Autodesk Fusion 360 part; units mm, degrees
(part 13 of 15)
  spline S115 degree 5 poles (45.7907, -108.2568) (45.7949, -108.2665) (45.806, -108.2927) (45.8241, -108.3354) (45.849, -108.3946) (45.8806, -108.4705) (45.9146, -108.5534) (45.9483, -108.6365) (45.9816, -108.7198) (46.0145, -108.8033) (46.0471, -108.8871) (46.0794, -108.971) (46.1114, -109.0551) (46.143, -109.1395) (46.1743, -109.224) (46.2052, -109.3087) (46.2359, -109.3936) (46.2662, -109.4787) (46.2962, -109.564) (46.3259, -109.6495) (46.3553, -109.7351) (46.3844, -109.8209) (46.4132, -109.9069) (46.4417, -109.9931) (46.4699, -110.0794) (46.4977, -110.1659) (46.5253, -110.2526) (46.5526, -110.3394) (46.5796, -110.4264) (46.6063, -110.5136) (46.6328, -110.6009) (46.6589, -110.6884) (46.6848, -110.776) (46.7103, -110.8637) (46.7356, -110.9517) (46.7606, -111.0397) (46.7854, -111.128) (46.8098, -111.2163) (46.834, -111.3048) (46.8579, -111.3935) (46.8816, -111.4823) (46.9049, -111.5712) (46.928, -111.6603) (46.9463, -111.7317) (46.9599, -111.7853) (46.9689, -111.821) (46.9733, -111.8389) knots 0.405839 0.405839 0.405839 0.405839 0.405839 0.405839 0.414286 0.428571 0.442857 0.457143 0.471429 0.485714 0.5 0.514286 0.528571 0.542857 0.557143 0.571429 0.585714 0.6 0.614286 0.628571 0.642857 0.657143 0.671429 0.685714 0.7 0.714286 0.728571 0.742857 0.757143 0.771429 0.785714 0.8 0.814286 0.828571 0.842857 0.857143 0.871429 0.885714 0.9 0.914286 0.928571 0.942857 0.957143 0.971429 0.985714 1 1 1 1 1 1
  arc A115 (45.9144, -112.6316) -> (46.9733, -111.8389) centre (2.0032, -52.8695) ccw
  spline S116 degree 5 poles (45.9144, -112.6316) (45.8985, -112.6223) (45.8667, -112.6036) (45.8191, -112.5754) (45.7558, -112.5378) (45.6769, -112.4906) (45.5981, -112.4431) (45.5196, -112.3954) (45.4412, -112.3475) (45.3631, -112.2993) (45.2852, -112.251) (45.2075, -112.2024) (45.1301, -112.1536) (45.0529, -112.1045) (44.9758, -112.0553) (44.8991, -112.0058) (44.8225, -111.956) (44.7462, -111.9061) (44.6701, -111.8559) (44.5942, -111.8055) (44.5186, -111.7548) (44.4432, -111.7039) (44.3681, -111.6528) (44.2932, -111.6015) (44.2185, -111.5499) (44.1441, -111.498) (44.07, -111.4459) (43.9961, -111.3936) (43.9224, -111.341) (43.8491, -111.2882) (43.776, -111.2351) (43.7031, -111.1818) (43.6306, -111.1282) (43.5583, -111.0744) (43.4863, -111.0203) (43.4145, -110.9659) (43.3431, -110.9113) (43.2719, -110.8564) (43.2011, -110.8012) (43.1305, -110.7458) (43.0603, -110.6901) (42.9903, -110.6341) (42.9264, -110.5825) (42.8766, -110.5419) (42.8407, -110.5125) (42.8188, -110.4944) (42.8106, -110.4877) knots -1 -1 -1 -1 -1 -1 -0.985714 -0.971429 -0.957143 -0.942857 -0.928571 -0.914286 -0.9 -0.885714 -0.871429 -0.857143 -0.842857 -0.828571 -0.814286 -0.8 -0.785714 -0.771429 -0.757143 -0.742857 -0.728571 -0.714286 -0.7 -0.685714 -0.671429 -0.657143 -0.642857 -0.628571 -0.614286 -0.6 -0.585714 -0.571429 -0.557143 -0.542857 -0.528571 -0.514286 -0.5 -0.485714 -0.471429 -0.457143 -0.442857 -0.428571 -0.414286 -0.405839 -0.405839 -0.405839 -0.405839 -0.405839 -0.405839
  arc A116 (41.7279, -111.2395) -> (42.8106, -110.4877) centre (2.0032, -52.8695) ccw
  spline S117 degree 5 poles (41.7279, -111.2395) (41.7313, -111.2494) (41.7406, -111.2763) (41.7556, -111.3202) (41.7762, -111.381) (41.8023, -111.459) (41.8303, -111.5441) (41.8579, -111.6294) (41.8852, -111.7149) (41.9121, -111.8005) (41.9387, -111.8864) (41.9649, -111.9724) (41.9907, -112.0586) (42.0163, -112.145) (42.0414, -112.2316) (42.0663, -112.3183) (42.0908, -112.4051) (42.115, -112.4922) (42.1388, -112.5794) (42.1624, -112.6668) (42.1856, -112.7543) (42.2085, -112.842) (42.231, -112.9298) (42.2533, -113.0178) (42.2753, -113.1059) (42.2969, -113.1942) (42.3182, -113.2826) (42.3393, -113.3711) (42.36, -113.4598) (42.3804, -113.5487) (42.4005, -113.6376) (42.4204, -113.7267) (42.4399, -113.816) (42.4592, -113.9054) (42.4781, -113.9949) (42.4968, -114.0845) (42.5152, -114.1742) (42.5332, -114.2641) (42.5511, -114.3541) (42.5686, -114.4443) (42.5858, -114.5345) (42.6028, -114.6249) (42.6195, -114.7154) (42.6326, -114.7879) (42.6423, -114.8423) (42.6487, -114.8786) (42.6519, -114.8968) knots 0.405839 0.405839 0.405839 0.405839 0.405839 0.405839 0.414286 0.428571 0.442857 0.457143 0.471429 0.485714 0.5 0.514286 0.528571 0.542857 0.557143 0.571429 0.585714 0.6 0.614286 0.628571 0.642857 0.657143 0.671429 0.685714 0.7 0.714286 0.728571 0.742857 0.757143 0.771429 0.785714 0.8 0.814286 0.828571 0.842857 0.857143 0.871429 0.885714 0.9 0.914286 0.928571 0.942857 0.957143 0.971429 0.985714 1 1 1 1 1 1
  arc A117 (41.5391, -115.6119) -> (42.6519, -114.8968) centre (2.0032, -52.8695) ccw
  spline S118 degree 5 poles (41.5391, -115.6119) (41.524, -115.6015) (41.4936, -115.5806) (41.4481, -115.5491) (41.3876, -115.5071) (41.3123, -115.4543) (41.2371, -115.4013) (41.1622, -115.3481) (41.0875, -115.2947) (41.013, -115.2412) (40.9387, -115.1874) (40.8647, -115.1334) (40.7909, -115.0791) (40.7174, -115.0247) (40.6441, -114.9701) (40.571, -114.9152) (40.4982, -114.8602) (40.4256, -114.8049) (40.3533, -114.7494) (40.2812, -114.6937) (40.2094, -114.6378) (40.1379, -114.5817) (40.0666, -114.5253) (39.9955, -114.4687) (39.9247, -114.412) (39.8542, -114.3549) (39.784, -114.2977) (39.714, -114.2402) (39.6443, -114.1825) (39.5749, -114.1246) (39.5058, -114.0664) (39.4369, -114.008) (39.3684, -113.9494) (39.3001, -113.8906) (39.2321, -113.8315) (39.1645, -113.7721) (39.0971, -113.7126) (39.03, -113.6527) (38.9633, -113.5927) (38.8969, -113.5323) (38.8308, -113.4718) (38.765, -113.4109) (38.7049, -113.3549) (38.6581, -113.3108) (38.6245, -113.279) (38.6038, -113.2594) (38.5962, -113.2521) knots -1 -1 -1 -1 -1 -1 -0.985714 -0.971429 -0.957143 -0.942857 -0.928571 -0.914286 -0.9 -0.885714 -0.871429 -0.857143 -0.842857 -0.828571 -0.814286 -0.8 -0.785714 -0.771429 -0.757143 -0.742857 -0.728571 -0.714286 -0.7 -0.685714 -0.671429 -0.657143 -0.642857 -0.628571 -0.614286 -0.6 -0.585714 -0.571429 -0.557143 -0.542857 -0.528571 -0.514286 -0.5 -0.485714 -0.471429 -0.457143 -0.442857 -0.428571 -0.414286 -0.405839 -0.405839 -0.405839 -0.405839 -0.405839 -0.405839
  arc A118 (37.4626, -113.9247) -> (38.5962, -113.2521) centre (2.0032, -52.8695) ccw
  spline S119 degree 5 poles (37.4626, -113.9247) (37.4653, -113.9349) (37.4726, -113.9624) (37.4845, -114.0072) (37.5007, -114.0693) (37.5211, -114.149) (37.543, -114.2358) (37.5645, -114.3229) (37.5856, -114.4101) (37.6063, -114.4975) (37.6267, -114.585) (37.6467, -114.6727) (37.6663, -114.7605) (37.6856, -114.8485) (37.7046, -114.9366) (37.7232, -115.0249) (37.7414, -115.1133) (37.7593, -115.2018) (37.7769, -115.2905) (37.7942, -115.3793) (37.8111, -115.4683) (37.8276, -115.5574) (37.8439, -115.6466) (37.8598, -115.7359) (37.8754, -115.8254) (37.8907, -115.915) (37.9057, -116.0047) (37.9204, -116.0945) (37.9347, -116.1845) (37.9487, -116.2745) (37.9625, -116.3647) (37.9759, -116.455) (37.989, -116.5454) (38.0018, -116.6359) (38.0144, -116.7266) (38.0266, -116.8173) (38.0385, -116.9081) (38.0501, -116.9991) (38.0615, -117.0901) (38.0725, -117.1813) (38.0833, -117.2726) (38.0938, -117.3639) (38.1039, -117.4554) (38.1119, -117.5286) (38.1177, -117.5836) (38.1215, -117.6203) (38.1234, -117.6386) knots 0.405839 0.405839 0.405839 0.405839 0.405839 0.405839 0.414286 0.428571 0.442857 0.457143 0.471429 0.485714 0.5 0.514286 0.528571 0.542857 0.557143 0.571429 0.585714 0.6 0.614286 0.628571 0.642857 0.657143 0.671429 0.685714 0.7 0.714286 0.728571 0.742857 0.757143 0.771429 0.785714 0.8 0.814286 0.828571 0.842857 0.857143 0.871429 0.885714 0.9 0.914286 0.928571 0.942857 0.957143 0.971429 0.985714 1 1 1 1 1 1
  arc A119 (36.9624, -118.2725) -> (38.1234, -117.6386) centre (2.0032, -52.8695) ccw
  spline S120 degree 5 poles (36.9624, -118.2725) (36.948, -118.261) (36.9192, -118.238) (36.8761, -118.2034) (36.8188, -118.1571) (36.7474, -118.0991) (36.6762, -118.0409) (36.6052, -117.9825) (36.5345, -117.9239) (36.464, -117.8652) (36.3938, -117.8062) (36.3238, -117.7471) (36.2541, -117.6877) (36.1846, -117.6282) (36.1154, -117.5685) (36.0465, -117.5086) (35.9778, -117.4484) (35.9093, -117.3881) (35.8411, -117.3276) (35.7732, -117.2669) (35.7056, -117.206) (35.6382, -117.1449) (35.5711, -117.0836) (35.5043, -117.0221) (35.4377, -116.9604) (35.3715, -116.8985) (35.3055, -116.8364) (35.2398, -116.7741) (35.1744, -116.7116) (35.1093, -116.6489) (35.0445, -116.5859) (34.98, -116.5228) (34.9158, -116.4594) (34.8519, -116.3958) (34.7883, -116.332) (34.725, -116.268) (34.6621, -116.2038) (34.5995, -116.1393) (34.5372, -116.0746) (34.4752, -116.0097) (34.4136, -115.9446) (34.3524, -115.8792) (34.2964, -115.819) (34.2529, -115.7718) (34.2216, -115.7376) (34.2024, -115.7166) (34.1953, -115.7087) knots -1 -1 -1 -1 -1 -1 -0.985714 -0.971429 -0.957143 -0.942857 -0.928571 -0.914286 -0.9 -0.885714 -0.871429 -0.857143 -0.842857 -0.828571 -0.814286 -0.8 -0.785714 -0.771429 -0.757143 -0.742857 -0.728571 -0.714286 -0.7 -0.685714 -0.671429 -0.657143 -0.642857 -0.628571 -0.614286 -0.6 -0.585714 -0.571429 -0.557143 -0.542857 -0.528571 -0.514286 -0.5 -0.485714 -0.471429 -0.457143 -0.442857 -0.428571 -0.414286 -0.405839 -0.405839 -0.405839 -0.405839 -0.405839 -0.405839
  arc A120 (33.0166, -116.2987) -> (34.1953, -115.7087) centre (2.0032, -52.8695) ccw
  spline S121 degree 5 poles (33.0166, -116.2987) (33.0186, -116.3091) (33.024, -116.3371) (33.0326, -116.3826) (33.0443, -116.4458) (33.059, -116.5266) (33.0746, -116.6149) (33.0898, -116.7032) (33.1047, -116.7917) (33.1191, -116.8803) (33.1332, -116.9691) (33.1469, -117.058) (33.1602, -117.147) (33.1732, -117.2361) (33.1858, -117.3254) (33.1981, -117.4147) (33.21, -117.5042) (33.2215, -117.5938) (33.2327, -117.6835) (33.2436, -117.7734) (33.2541, -117.8633) (33.2643, -117.9533) (33.2741, -118.0435) (33.2836, -118.1337) (33.2928, -118.2241) (33.3017, -118.3145) (33.3102, -118.4051) (33.3184, -118.4957) (33.3263, -118.5865) (33.3339, -118.6773) (33.3412, -118.7682) (33.3481, -118.8593) (33.3547, -118.9504) (33.3611, -119.0416) (33.3671, -119.1329) (33.3728, -119.2242) (33.3782, -119.3157) (33.3833, -119.4073) (33.3882, -119.4989) (33.3927, -119.5906) (33.3969, -119.6824) (33.4008, -119.7743) (33.4045, -119.8662) (33.4071, -119.9398) (33.409, -119.9951) (33.4102, -120.0319) (33.4108, -120.0504) knots 0.405839 0.405839 0.405839 0.405839 0.405839 0.405839 0.414286 0.428571 0.442857 0.457143 0.471429 0.485714 0.5 0.514286 0.528571 0.542857 0.557143 0.571429 0.585714 0.6 0.614286 0.628571 0.642857 0.657143 0.671429 0.685714 0.7 0.714286 0.728571 0.742857 0.757143 0.771429 0.785714 0.8 0.814286 0.828571 0.842857 0.857143 0.871429 0.885714 0.9 0.914286 0.928571 0.942857 0.957143 0.971429 0.985714 1 1 1 1 1 1
  arc A121 (32.2075, -120.5999) -> (33.4108, -120.0504) centre (2.0032, -52.8695) ccw
  spline S122 degree 5 poles (32.2075, -120.5999) (32.194, -120.5873) (32.1669, -120.5623) (32.1264, -120.5247) (32.0725, -120.4745) (32.0054, -120.4115) (31.9385, -120.3484) (31.8719, -120.2851) (31.8056, -120.2216) (31.7395, -120.158) (31.6737, -120.0942) (31.6081, -120.0302) (31.5428, -119.966) (31.4777, -119.9017) (31.4129, -119.8372) (31.3484, -119.7725) (31.2842, -119.7076) (31.2202, -119.6426) (31.1565, -119.5774) (31.0931, -119.512) (31.03, -119.4464) (30.9672, -119.3807) (30.9046, -119.3147) (30.8423, -119.2486) (30.7804, -119.1823) (30.7187, -119.1159) (30.6573, -119.0492) (30.5962, -118.9824) (30.5354, -118.9153) (30.475, -118.8481) (30.4148, -118.7807) (30.355, -118.7131) (30.2955, -118.6453) (30.2363, -118.5774) (30.1774, -118.5092) (30.1189, -118.4408) (30.0607, -118.3723) (30.0028, -118.3035) (29.9453, -118.2346) (29.8881, -118.1654) (29.8313, -118.096) (29.7749, -118.0265) (29.7234, -117.9624) (29.6833, -117.9122) (29.6545, -117.8758) (29.6369, -117.8535) (29.6304, -117.8452) knots -1 -1 -1 -1 -1 -1 -0.985714 -0.971429 -0.957143 -0.942857 -0.928571 -0.914286 -0.9 -0.885714 -0.871429 -0.857143 -0.842857 -0.828571 -0.814286 -0.8 -0.785714 -0.771429 -0.757143 -0.742857 -0.728571 -0.714286 -0.7 -0.685714 -0.671429 -0.657143 -0.642857 -0.628571 -0.614286 -0.6 -0.585714 -0.571429 -0.557143 -0.542857 -0.528571 -0.514286 -0.5 -0.485714 -0.471429 -0.457143 -0.442857 -0.428571 -0.414286 -0.405839 -0.405839 -0.405839 -0.405839 -0.405839 -0.405839
  arc A122 (28.4126, -118.3496) -> (29.6304, -117.8452) centre (2.0032, -52.8695) ccw
  spline S123 degree 5 poles (28.4126, -118.3496) (28.4139, -118.3601) (28.4172, -118.3884) (28.4225, -118.4344) (28.4298, -118.4982) (28.4386, -118.58) (28.4479, -118.6691) (28.4568, -118.7583) (28.4653, -118.8476) (28.4734, -118.937) (28.4811, -119.0266) (28.4884, -119.1162) (28.4953, -119.2059) (28.5019, -119.2958) (28.5081, -119.3857) (28.514, -119.4757) (28.5195, -119.5658) (28.5246, -119.656) (28.5294, -119.7463) (28.5338, -119.8366) (28.5379, -119.9271) (28.5416, -120.0176) (28.545, -120.1083) (28.548, -120.199) (28.5507, -120.2897) (28.5531, -120.3806) (28.5552, -120.4715) (28.5569, -120.5625) (28.5583, -120.6536) (28.5594, -120.7447) (28.5601, -120.836) (28.5606, -120.9272) (28.5607, -121.0186) (28.5605, -121.11) (28.56, -121.2015) (28.5592, -121.2931) (28.5581, -121.3847) (28.5566, -121.4764) (28.5549, -121.5681) (28.5529, -121.6599) (28.5505, -121.7518) (28.5479, -121.8437) (28.545, -121.9356) (28.5424, -122.0093) (28.5403, -122.0645) (28.5389, -122.1014) (28.5381, -122.1198) knots 0.405839 0.405839 0.405839 0.405839 0.405839 0.405839 0.414286 0.428571 0.442857 0.457143 0.471429 0.485714 0.5 0.514286 0.528571 0.542857 0.557143 0.571429 0.585714 0.6 0.614286 0.628571 0.642857 0.657143 0.671429 0.685714 0.7 0.714286 0.728571 0.742857 0.757143 0.771429 0.785714 0.8 0.814286 0.828571 0.842857 0.857143 0.871429 0.885714 0.9 0.914286 0.928571 0.942857 0.957143 0.971429 0.985714 1 1 1 1 1 1
  arc A123 (27.2988, -122.582) -> (28.5381, -122.1198) centre (2.0032, -52.8695) ccw
  spline S124 degree 5 poles (27.2988, -122.582) (27.2861, -122.5686) (27.2609, -122.5417) (27.2232, -122.5013) (27.173, -122.4474) (27.1106, -122.3798) (27.0484, -122.312) (26.9865, -122.2441) (26.9248, -122.1761) (26.8634, -122.1079) (26.8023, -122.0395) (26.7415, -121.971) (26.6809, -121.9024) (26.6206, -121.8336) (26.5606, -121.7646) (26.5009, -121.6955) (26.4414, -121.6262) (26.3822, -121.5568) (26.3234, -121.4872) (26.2648, -121.4174) (26.2065, -121.3475) (26.1485, -121.2775) (26.0908, -121.2072) (26.0334, -121.1369) (25.9763, -121.0663) (25.9195, -120.9956) (25.8631, -120.9247) (25.8069, -120.8537) (25.7511, -120.7825) (25.6956, -120.7112) (25.6404, -120.6396) (25.5855, -120.5679) (25.531, -120.4961) (25.4768, -120.4241) (25.4229, -120.3519) (25.3694, -120.2795) (25.3163, -120.207) (25.2635, -120.1343) (25.211, -120.0614) (25.1589, -119.9883) (25.1072, -119.9151) (25.0559, -119.8417) (25.0091, -119.7741) (24.9727, -119.7211) (24.9466, -119.6828) (24.9306, -119.6593) (24.9247, -119.6505) knots -1 -1 -1 -1 -1 -1 -0.985714 -0.971429 -0.957143 -0.942857 -0.928571 -0.914286 -0.9 -0.885714 -0.871429 -0.857143 -0.842857 -0.828571 -0.814286 -0.8 -0.785714 -0.771429 -0.757143 -0.742857 -0.728571 -0.714286 -0.7 -0.685714 -0.671429 -0.657143 -0.642857 -0.628571 -0.614286 -0.6 -0.585714 -0.571429 -0.557143 -0.542857 -0.528571 -0.514286 -0.5 -0.485714 -0.471429 -0.457143 -0.442857 -0.428571 -0.414286 -0.405839 -0.405839 -0.405839 -0.405839 -0.405839 -0.405839
  arc A124 (23.674, -120.0668) -> (24.9247, -119.6505) centre (2.0032, -52.8695) ccw
  spline S125 degree 5 poles (23.674, -120.0668) (23.6745, -120.0774) (23.6758, -120.1058) (23.6779, -120.1521) (23.6805, -120.2163) (23.6836, -120.2984) (23.6864, -120.388) (23.6889, -120.4776) (23.691, -120.5673) (23.6927, -120.6571) (23.694, -120.7469) (23.6949, -120.8368) (23.6955, -120.9268) (23.6956, -121.0169) (23.6954, -121.107) (23.6948, -121.1972) (23.6938, -121.2875) (23.6925, -121.3778) (23.6908, -121.4682) (23.6888, -121.5587) (23.6864, -121.6492) (23.6837, -121.7398) (23.6806, -121.8304) (23.6772, -121.9211) (23.6734, -122.0118) (23.6693, -122.1026) (23.6649, -122.1935) (23.6601, -122.2844) (23.655, -122.3753) (23.6496, -122.4663) (23.6438, -122.5573) (23.6377, -122.6484) (23.6313, -122.7396) (23.6246, -122.8307) (23.6176, -122.9219) (23.6102, -123.0132) (23.6026, -123.1045) (23.5946, -123.1959) (23.5864, -123.2872) (23.5778, -123.3787) (23.5689, -123.4701) (23.5597, -123.5616) (23.5502, -123.6531) (23.5424, -123.7264) (23.5364, -123.7813) (23.5323, -123.818) (23.5303, -123.8363) knots 0.405839 0.405839 0.405839 0.405839 0.405839 0.405839 0.414286 0.428571 0.442857 0.457143 0.471429 0.485714 0.5 0.514286 0.528571 0.542857 0.557143 0.571429 0.585714 0.6 0.614286 0.628571 0.642857 0.657143 0.671429 0.685714 0.7 0.714286 0.728571 0.742857 0.757143 0.771429 0.785714 0.8 0.814286 0.828571 0.842857 0.857143 0.871429 0.885714 0.9 0.914286 0.928571 0.942857 0.957143 0.971429 0.985714 1 1 1 1 1 1
  arc A125 (22.2611, -124.209) -> (23.5303, -123.8363) centre (2.0032, -52.8695) ccw
  spline S126 degree 5 poles (22.2611, -124.209) (22.2494, -124.1947) (22.2262, -124.166) (22.1914, -124.1231) (22.1453, -124.0657) (22.0878, -123.9938) (22.0306, -123.9218) (21.9737, -123.8497) (21.917, -123.7774) (21.8607, -123.705) (21.8046, -123.6325) (21.7488, -123.5598) (21.6933, -123.487) (21.638, -123.414) (21.5831, -123.341) (21.5284, -123.2678) (21.4741, -123.1944) (21.42, -123.1209) (21.3663, -123.0473) (21.3128, -122.9736) (21.2597, -122.8997) (21.2068, -122.8257) (21.1543, -122.7515) (21.102, -122.6772) (21.0501, -122.6028) (20.9985, -122.5282) (20.9473, -122.4535) (20.8963, -122.3786) (20.8457, -122.3036) (20.7954, -122.2285) (20.7455, -122.1532) (20.6959, -122.0778) (20.6466, -122.0022) (20.5977, -121.9265) (20.5491, -121.8507) (20.5009, -121.7747) (20.4531, -121.6985) (20.4056, -121.6222) (20.3585, -121.5458) (20.3117, -121.4692) (20.2654, -121.3925) (20.2194, -121.3156) (20.1775, -121.2448) (20.145, -121.1894) (20.1217, -121.1493) (20.1075, -121.1247) (20.1022, -121.1156) knots -1 -1 -1 -1 -1 -1 -0.985714 -0.971429 -0.957143 -0.942857 -0.928571 -0.914286 -0.9 -0.885714 -0.871429 -0.857143 -0.842857 -0.828571 -0.814286 -0.8 -0.785714 -0.771429 -0.757143 -0.742857 -0.728571 -0.714286 -0.7 -0.685714 -0.671429 -0.657143 -0.642857 -0.628571 -0.614286 -0.6 -0.585714 -0.571429 -0.557143 -0.542857 -0.528571 -0.514286 -0.5 -0.485714 -0.471429 -0.457143 -0.442857 -0.428571 -0.414286 -0.405839 -0.405839 -0.405839 -0.405839 -0.405839 -0.405839
  arc A126 (18.825, -121.4416) -> (20.1022, -121.1156) centre (2.0032, -52.8695) ccw
  spline S127 degree 5 poles (18.825, -121.4416) (18.8248, -121.4521) (18.824, -121.4806) (18.8228, -121.5269) (18.8208, -121.5911) (18.818, -121.6733) (18.8145, -121.7628) (18.8106, -121.8524) (18.8063, -121.942) (18.8015, -122.0317) (18.7964, -122.1214) (18.7909, -122.2111) (18.785, -122.3009) (18.7788, -122.3908) (18.7721, -122.4807) (18.7651, -122.5706) (18.7577, -122.6606) (18.7499, -122.7506) (18.7418, -122.8406) (18.7333, -122.9307) (18.7245, -123.0208) (18.7153, -123.111) (18.7057, -123.2012) (18.6959, -123.2914) (18.6856, -123.3816) (18.6751, -123.4719) (18.6641, -123.5622) (18.6529, -123.6525) (18.6413, -123.7428) (18.6294, -123.8332) (18.6172, -123.9236) (18.6046, -124.014) (18.5918, -124.1045) (18.5786, -124.1949) (18.565, -124.2854) (18.5512, -124.3759) (18.537, -124.4664) (18.5226, -124.557) (18.5078, -124.6475) (18.4927, -124.7381) (18.4774, -124.8287) (18.4617, -124.9193) (18.4457, -125.0099) (18.4326, -125.0824) (18.4227, -125.1368) (18.4161, -125.1731) (18.4127, -125.1912) knots 0.405839 0.405839 0.405839 0.405839 0.405839 0.405839 0.414286 0.428571 0.442857 0.457143 0.471429 0.485714 0.5 0.514286 0.528571 0.542857 0.557143 0.571429 0.585714 0.6 0.614286 0.628571 0.642857 0.657143 0.671429 0.685714 0.7 0.714286 0.728571 0.742857 0.757143 0.771429 0.785714 0.8 0.814286 0.828571 0.842857 0.857143 0.871429 0.885714 0.9 0.914286 0.928571 0.942857 0.957143 0.971429 0.985714 1 1 1 1 1 1
  arc A127 (17.1202, -125.4724) -> (18.4127, -125.1912) centre (2.0032, -52.8695) ccw
  spline S128 degree 5 poles (17.1202, -125.4724) (17.1096, -125.4573) (17.0884, -125.4271) (17.0568, -125.3817) (17.0149, -125.3212) (16.9627, -125.2454) (16.9108, -125.1695) (16.8591, -125.0935) (16.8078, -125.0174) (16.7567, -124.9411) (16.706, -124.8648) (16.6555, -124.7883) (16.6053, -124.7117) (16.5554, -124.635) (16.5058, -124.5582) (16.4565, -124.4813) (16.4076, -124.4043) (16.3589, -124.3271) (16.3105, -124.2499) (16.2624, -124.1725) (16.2147, -124.095) (16.1673, -124.0174) (16.1202, -123.9397) (16.0734, -123.8618) (16.0269, -123.7839) (15.9808, -123.7058) (15.9349, -123.6277) (15.8895, -123.5494) (15.8443, -123.4709) (15.7995, -123.3924) (15.7551, -123.3138) (15.711, -123.235) (15.6672, -123.1561) (15.6238, -123.0771) (15.5808, -122.998) (15.5381, -122.9187) (15.4958, -122.8394) (15.4539, -122.7599) (15.4124, -122.6803) (15.3712, -122.6005) (15.3305, -122.5207) (15.2901, -122.4407) (15.2534, -122.3672) (15.2249, -122.3096) (15.2045, -122.2679) (15.1921, -122.2424) (15.1874, -122.2329) knots -1 -1 -1 -1 -1 -1 -0.985714 -0.971429 -0.957143 -0.942857 -0.928571 -0.914286 -0.9 -0.885714 -0.871429 -0.857143 -0.842857 -0.828571 -0.814286 -0.8 -0.785714 -0.771429 -0.757143 -0.742857 -0.728571 -0.714286 -0.7 -0.685714 -0.671429 -0.657143 -0.642857 -0.628571 -0.614286 -0.6 -0.585714 -0.571429 -0.557143 -0.542857 -0.528571 -0.514286 -0.5 -0.485714 -0.471429 -0.457143 -0.442857 -0.428571 -0.414286 -0.405839 -0.405839 -0.405839 -0.405839 -0.405839 -0.405839
  arc A128 (13.8903, -122.4669) -> (15.1874, -122.2329) centre (2.0032, -52.8695) ccw
  spline S129 degree 5 poles (13.8903, -122.4669) (13.8893, -122.4774) (13.8865, -122.5057) (13.882, -122.5519) (13.8754, -122.6158) (13.8667, -122.6975) (13.8569, -122.7866) (13.8466, -122.8756) (13.8359, -122.9647) (13.8248, -123.0538) (13.8133, -123.1429) (13.8014, -123.2321) (13.7891, -123.3212) (13.7764, -123.4104) (13.7634, -123.4996) (13.7499, -123.5888) (13.7361, -123.678) (13.722, -123.7672) (13.7075, -123.8565) (13.6926, -123.9457) (13.6773, -124.035) (13.6617, -124.1242) (13.6458, -124.2135) (13.6295, -124.3028) (13.6128, -124.3921) (13.5959, -124.4813) (13.5785, -124.5706) (13.5609, -124.6599) (13.5429, -124.7492) (13.5246, -124.8385) (13.5059, -124.9278) (13.4869, -125.0171) (13.4676, -125.1064) (13.448, -125.1957) (13.4281, -125.285) (13.4078, -125.3742) (13.3873, -125.4635) (13.3664, -125.5528) (13.3452, -125.6421) (13.3237, -125.7314) (13.3019, -125.8206) (13.2798, -125.9099) (13.2573, -125.9991) (13.2392, -126.0705) (13.2254, -126.1241) (13.2162, -126.1597) (13.2115, -126.1776) knots 0.405839 0.405839 0.405839 0.405839 0.405839 0.405839 0.414286 0.428571 0.442857 0.457143 0.471429 0.485714 0.5 0.514286 0.528571 0.542857 0.557143 0.571429 0.585714 0.6 0.614286 0.628571 0.642857 0.657143 0.671429 0.685714 0.7 0.714286 0.728571 0.742857 0.757143 0.771429 0.785714 0.8 0.814286 0.828571 0.842857 0.857143 0.871429 0.885714 0.9 0.914286 0.928571 0.942857 0.957143 0.971429 0.985714 1 1 1 1 1 1
  arc A129 (11.9022, -126.3658) -> (13.2115, -126.1776) centre (2.0032, -52.8695) ccw
  spline S130 degree 5 poles (11.9022, -126.3658) (11.8927, -126.35) (11.8738, -126.3184) (11.8455, -126.2709) (11.808, -126.2075) (11.7613, -126.1282) (11.7149, -126.0488) (11.6689, -125.9693) (11.6231, -125.8897) (11.5776, -125.81) (11.5324, -125.7302) (11.4875, -125.6503) (11.4429, -125.5704) (11.3986, -125.4903) (11.3547, -125.4102) (11.311, -125.3299) (11.2676, -125.2496) (11.2246, -125.1692) (11.1818, -125.0887) (11.1394, -125.0081) (11.0973, -124.9274) (11.0555, -124.8466) (11.0141, -124.7657) (10.973, -124.6847) (10.9322, -124.6037) (10.8917, -124.5225) (10.8516, -124.4412) (10.8118, -124.3599) (10.7724, -124.2785) (10.7333, -124.1969) (10.6946, -124.1153) (10.6562, -124.0336) (10.6182, -123.9518) (10.5806, -123.8699) (10.5433, -123.7879) (10.5064, -123.7058) (10.4699, -123.6236) (10.4337, -123.5414) (10.398, -123.459) (10.3626, -123.3765) (10.3276, -123.294) (10.2931, -123.2113) (10.2617, -123.1353) (10.2374, -123.0759) (10.2201, -123.0329) (10.2095, -123.0065) (10.2055, -122.9967) knots -1 -1 -1 -1 -1 -1 -0.985714 -0.971429 -0.957143 -0.942857 -0.928571 -0.914286 -0.9 -0.885714 -0.871429 -0.857143 -0.842857 -0.828571 -0.814286 -0.8 -0.785714 -0.771429 -0.757143 -0.742857 -0.728571 -0.714286 -0.7 -0.685714 -0.671429 -0.657143 -0.642857 -0.628571 -0.614286 -0.6 -0.585714 -0.571429 -0.557143 -0.542857 -0.528571 -0.514286 -0.5 -0.485714 -0.471429 -0.457143 -0.442857 -0.428571 -0.414286 -0.405839 -0.405839 -0.405839 -0.405839 -0.405839 -0.405839
  arc A130 (8.895, -123.1376) -> (10.2055, -122.9967) centre (2.0032, -52.8695) ccw
  spline S131 degree 5 poles (8.895, -123.1376) (8.8932, -123.148) (8.8884, -123.1761) (8.8806, -123.2217) (8.8695, -123.285) (8.855, -123.3659) (8.8388, -123.454) (8.8222, -123.5421) (8.8052, -123.6302) (8.7878, -123.7183) (8.7699, -123.8064) (8.7517, -123.8945) (8.7331, -123.9825) (8.7141, -124.0706) (8.6947, -124.1586) (8.675, -124.2466) (8.6548, -124.3346) (8.6343, -124.4226) (8.6135, -124.5106) (8.5923, -124.5985) (8.5707, -124.6865) (8.5488, -124.7744) (8.5265, -124.8623) (8.5039, -124.9502) (8.4809, -125.038) (8.4576, -125.1259) (8.4339, -125.2137) (8.41, -125.3015) (8.3856, -125.3893) (8.361, -125.4771) (8.336, -125.5648) (8.3107, -125.6525) (8.2851, -125.7402) (8.2592, -125.8279) (8.2329, -125.9155) (8.2063, -126.0031) (8.1794, -126.0907) (8.1522, -126.1783) (8.1247, -126.2658) (8.0969, -126.3533) (8.0688, -126.4408) (8.0404, -126.5282) (8.0117, -126.6157) (7.9884, -126.6856) (7.9709, -126.738) (7.9591, -126.7729) (7.9532, -126.7904) knots 0.405839 0.405839 0.405839 0.405839 0.405839 0.405839 0.414286 0.428571 0.442857 0.457143 0.471429 0.485714 0.5 0.514286 0.528571 0.542857 0.557143 0.571429 0.585714 0.6 0.614286 0.628571 0.642857 0.657143 0.671429 0.685714 0.7 0.714286 0.728571 0.742857 0.757143 0.771429 0.785714 0.8 0.814286 0.828571 0.842857 0.857143 0.871429 0.885714 0.9 0.914286 0.928571 0.942857 0.957143 0.971429 0.985714 1 1 1 1 1 1
  arc A131 (6.6338, -126.8848) -> (7.9532, -126.7904) centre (2.0032, -52.8695) ccw
  spline S132 degree 5 poles (6.6338, -126.8848) (6.6255, -126.8683) (6.6089, -126.8354) (6.584, -126.786) (6.5511, -126.7201) (6.5102, -126.6377) (6.4697, -126.5552) (6.4294, -126.4726) (6.3894, -126.3899) (6.3497, -126.3072) (6.3103, -126.2244) (6.2712, -126.1415) (6.2325, -126.0586) (6.194, -125.9756) (6.1558, -125.8925) (6.118, -125.8093) (6.0805, -125.7261) (6.0433, -125.6428) (6.0064, -125.5595) (5.9698, -125.476) (5.9336, -125.3925) (5.8977, -125.309) (5.8621, -125.2253) (5.8269, -125.1416) (5.792, -125.0579) (5.7574, -124.974) (5.7232, -124.8901) (5.6893, -124.8062) (5.6558, -124.7221) (5.6227, -124.638) (5.5898, -124.5538) (5.5574, -124.4696) (5.5253, -124.3853) (5.4936, -124.3009) (5.4623, -124.2165) (5.4313, -124.132) (5.4008, -124.0474) (5.3706, -123.9627) (5.3408, -123.878) (5.3114, -123.7932) (5.2824, -123.7084) (5.2538, -123.6235) (5.228, -123.5455) (5.208, -123.4844) (5.1937, -123.4403) (5.185, -123.4132) (5.1818, -123.4032) knots -1 -1 -1 -1 -1 -1 -0.985714 -0.971429 -0.957143 -0.942857 -0.928571 -0.914286 -0.9 -0.885714 -0.871429 -0.857143 -0.842857 -0.828571 -0.814286 -0.8 -0.785714 -0.771429 -0.757143 -0.742857 -0.728571 -0.714286 -0.7 -0.685714 -0.671429 -0.657143 -0.642857 -0.628571 -0.614286 -0.6 -0.585714 -0.571429 -0.557143 -0.542857 -0.528571 -0.514286 -0.5 -0.485714 -0.471429 -0.457143 -0.442857 -0.428571 -0.414286 -0.405839 -0.405839 -0.405839 -0.405839 -0.405839 -0.405839
  arc A132 (3.8645, -123.4502) -> (5.1818, -123.4032) centre (2.0032, -52.8695) ccw
  spline S133 degree 5 poles (3.8645, -123.4502) (3.862, -123.4605) (3.8553, -123.4881) (3.8442, -123.5331) (3.8287, -123.5954) (3.8084, -123.6751) (3.786, -123.7619) (3.7631, -123.8485) (3.7398, -123.9352) (3.7162, -124.0218) (3.6921, -124.1084) (3.6676, -124.1949) (3.6428, -124.2814) (3.6176, -124.3679) (3.592, -124.4543) (3.566, -124.5407) (3.5396, -124.6271) (3.5129, -124.7134) (3.4858, -124.7996) (3.4584, -124.8858) (3.4306, -124.972) (3.4025, -125.0581) (3.374, -125.1442) (3.3451, -125.2303) (3.316, -125.3163) (3.2864, -125.4022) (3.2566, -125.4881) (3.2264, -125.574) (3.1959, -125.6598) (3.165, -125.7456) (3.1339, -125.8313) (3.1024, -125.917) (3.0706, -126.0027) (3.0384, -126.0883) (3.006, -126.1738) (2.9732, -126.2593) (2.9402, -126.3447) (2.9068, -126.4301) (2.8731, -126.5155) (2.8391, -126.6008) (2.8048, -126.686) (2.7702, -126.7712) (2.7354, -126.8564) (2.7072, -126.9245) (2.686, -126.9755) (2.6717, -127.0095) (2.6646, -127.0265) knots 0.405839 0.405839 0.405839 0.405839 0.405839 0.405839 0.414286 0.428571 0.442857 0.457143 0.471429 0.485714 0.5 0.514286 0.528571 0.542857 0.557143 0.571429 0.585714 0.6 0.614286 0.628571 0.642857 0.657143 0.671429 0.685714 0.7 0.714286 0.728571 0.742857 0.757143 0.771429 0.785714 0.8 0.814286 0.828571 0.842857 0.857143 0.871429 0.885714 0.9 0.914286 0.928571 0.942857 0.957143 0.971429 0.985714 1 1 1 1 1 1
  arc A133 (1.3418, -127.0265) -> (2.6646, -127.0265) centre (2.0032, -52.8695) ccw
  spline S134 degree 5 poles (1.3418, -127.0265) (1.3347, -127.0095) (1.3205, -126.9755) (1.2992, -126.9245) (1.2711, -126.8564) (1.2362, -126.7712) (1.2016, -126.686) (1.1673, -126.6008) (1.1333, -126.5155) (1.0996, -126.4301) (1.0663, -126.3447) (1.0332, -126.2593) (1.0004, -126.1738) (0.968, -126.0883) (0.9359, -126.0027) (0.904, -125.917) (0.8726, -125.8313) (0.8414, -125.7456) (0.8105, -125.6598) (0.78, -125.574) (0.7498, -125.4881) (0.72, -125.4022) (0.6905, -125.3163) (0.6613, -125.2303) (0.6325, -125.1442) (0.604, -125.0581) (0.5758, -124.972) (0.548, -124.8858) (0.5206, -124.7996) (0.4935, -124.7134) (0.4668, -124.6271) (0.4405, -124.5407) (0.4145, -124.4543) (0.3889, -124.3679) (0.3636, -124.2814) (0.3388, -124.1949) (0.3143, -124.1084) (0.2903, -124.0218) (0.2666, -123.9352) (0.2433, -123.8485) (0.2205, -123.7619) (0.198, -123.6751) (0.1778, -123.5954) (0.1622, -123.5331) (0.1511, -123.4881) (0.1444, -123.4605) (0.1419, -123.4502) knots -1 -1 -1 -1 -1 -1 -0.985714 -0.971429 -0.957143 -0.942857 -0.928571 -0.914286 -0.9 -0.885714 -0.871429 -0.857143 -0.842857 -0.828571 -0.814286 -0.8 -0.785714 -0.771429 -0.757143 -0.742857 -0.728571 -0.714286 -0.7 -0.685714 -0.671429 -0.657143 -0.642857 -0.628571 -0.614286 -0.6 -0.585714 -0.571429 -0.557143 -0.542857 -0.528571 -0.514286 -0.5 -0.485714 -0.471429 -0.457143 -0.442857 -0.428571 -0.414286 -0.405839 -0.405839 -0.405839 -0.405839 -0.405839 -0.405839
  arc A134 (-1.1754, -123.4032) -> (0.1419, -123.4502) centre (2.0032, -52.8695) ccw
  spline S135 degree 5 poles (-1.1754, -123.4032) (-1.1786, -123.4132) (-1.1873, -123.4403) (-1.2016, -123.4844) (-1.2215, -123.5455) (-1.2474, -123.6235) (-1.276, -123.7084) (-1.305, -123.7932) (-1.3344, -123.878) (-1.3641, -123.9627) (-1.3943, -124.0474) (-1.4249, -124.132) (-1.4559, -124.2165) (-1.4872, -124.3009) (-1.5189, -124.3853) (-1.551, -124.4696) (-1.5834, -124.5538) (-1.6162, -124.638) (-1.6494, -124.7221) (-1.6829, -124.8062) (-1.7168, -124.8901) (-1.751, -124.974) (-1.7855, -125.0579) (-1.8205, -125.1416) (-1.8557, -125.2253) (-1.8913, -125.309) (-1.9272, -125.3925) (-1.9634, -125.476) (-2, -125.5595) (-2.0368, -125.6428) (-2.074, -125.7261) (-2.1116, -125.8093) (-2.1494, -125.8925) (-2.1876, -125.9756) (-2.226, -126.0586) (-2.2648, -126.1415) (-2.3039, -126.2244) (-2.3433, -126.3072) (-2.383, -126.3899) (-2.4229, -126.4726) (-2.4632, -126.5552) (-2.5038, -126.6377) (-2.5447, -126.7201) (-2.5776, -126.786) (-2.6024, -126.8354) (-2.6191, -126.8683) (-2.6274, -126.8848) knots 0.405839 0.405839 0.405839 0.405839 0.405839 0.405839 0.414286 0.428571 0.442857 0.457143 0.471429 0.485714 0.5 0.514286 0.528571 0.542857 0.557143 0.571429 0.585714 0.6 0.614286 0.628571 0.642857 0.657143 0.671429 0.685714 0.7 0.714286 0.728571 0.742857 0.757143 0.771429 0.785714 0.8 0.814286 0.828571 0.842857 0.857143 0.871429 0.885714 0.9 0.914286 0.928571 0.942857 0.957143 0.971429 0.985714 1 1 1 1 1 1
  arc A135 (-3.9468, -126.7904) -> (-2.6274, -126.8848) centre (2.0032, -52.8695) ccw
  spline S136 degree 5 poles (-3.9468, -126.7904) (-3.9527, -126.7729) (-3.9645, -126.738) (-3.982, -126.6856) (-4.0052, -126.6157) (-4.034, -126.5282) (-4.0624, -126.4408) (-4.0905, -126.3533) (-4.1183, -126.2658) (-4.1458, -126.1783) (-4.173, -126.0907) (-4.1999, -126.0031) (-4.2265, -125.9155) (-4.2527, -125.8279) (-4.2787, -125.7402) (-4.3043, -125.6525) (-4.3296, -125.5648) (-4.3546, -125.4771) (-4.3792, -125.3893) (-4.4035, -125.3015) (-4.4275, -125.2137) (-4.4512, -125.1259) (-4.4745, -125.038) (-4.4974, -124.9502) (-4.5201, -124.8623) (-4.5423, -124.7744) (-4.5643, -124.6865) (-4.5858, -124.5985) (-4.6071, -124.5106) (-4.6279, -124.4226) (-4.6484, -124.3346) (-4.6685, -124.2466) (-4.6883, -124.1586) (-4.7077, -124.0706) (-4.7267, -123.9825) (-4.7453, -123.8945) (-4.7635, -123.8064) (-4.7813, -123.7183) (-4.7988, -123.6302) (-4.8158, -123.5421) (-4.8324, -123.454) (-4.8486, -123.3659) (-4.8631, -123.285) (-4.8742, -123.2217) (-4.882, -123.1761) (-4.8868, -123.148) (-4.8885, -123.1376) knots -1 -1 -1 -1 -1 -1 -0.985714 -0.971429 -0.957143 -0.942857 -0.928571 -0.914286 -0.9 -0.885714 -0.871429 -0.857143 -0.842857 -0.828571 -0.814286 -0.8 -0.785714 -0.771429 -0.757143 -0.742857 -0.728571 -0.714286 -0.7 -0.685714 -0.671429 -0.657143 -0.642857 -0.628571 -0.614286 -0.6 -0.585714 -0.571429 -0.557143 -0.542857 -0.528571 -0.514286 -0.5 -0.485714 -0.471429 -0.457143 -0.442857 -0.428571 -0.414286 -0.405839 -0.405839 -0.405839 -0.405839 -0.405839 -0.405839
  arc A136 (-6.1991, -122.9967) -> (-4.8885, -123.1376) centre (2.0032, -52.8695) ccw
  spline S137 degree 5 poles (-6.1991, -122.9967) (-6.203, -123.0065) (-6.2136, -123.0329) (-6.231, -123.0759) (-6.2553, -123.1353) (-6.2866, -123.2113) (-6.3212, -123.294) (-6.3562, -123.3765) (-6.3915, -123.459) (-6.4273, -123.5414) (-6.4634, -123.6236) (-6.5, -123.7058) (-6.5369, -123.7879) (-6.5742, -123.8699) (-6.6118, -123.9518) (-6.6498, -124.0336) (-6.6882, -124.1153) (-6.7269, -124.1969) (-6.766, -124.2785) (-6.8054, -124.3599) (-6.8452, -124.4412) (-6.8853, -124.5225) (-6.9258, -124.6037) (-6.9665, -124.6847) (-7.0077, -124.7657) (-7.0491, -124.8466) (-7.0909, -124.9274) (-7.133, -125.0081) (-7.1754, -125.0887) (-7.2181, -125.1692) (-7.2612, -125.2496) (-7.3046, -125.3299) (-7.3482, -125.4102) (-7.3922, -125.4903) (-7.4365, -125.5704) (-7.4811, -125.6503) (-7.526, -125.7302) (-7.5712, -125.81) (-7.6167, -125.8897) (-7.6624, -125.9693) (-7.7085, -126.0488) (-7.7549, -126.1282) (-7.8015, -126.2075) (-7.8391, -126.2709) (-7.8674, -126.3184) (-7.8863, -126.35) (-7.8958, -126.3658) knots 0.405839 0.405839 0.405839 0.405839 0.405839 0.405839 0.414286 0.428571 0.442857 0.457143 0.471429 0.485714 0.5 0.514286 0.528571 0.542857 0.557143 0.571429 0.585714 0.6 0.614286 0.628571 0.642857 0.657143 0.671429 0.685714 0.7 0.714286 0.728571 0.742857 0.757143 0.771429 0.785714 0.8 0.814286 0.828571 0.842857 0.857143 0.871429 0.885714 0.9 0.914286 0.928571 0.942857 0.957143 0.971429 0.985714 1 1 1 1 1 1
  arc A137 (-9.2051, -126.1776) -> (-7.8958, -126.3658) centre (2.0032, -52.8695) ccw
  spline S138 degree 5 poles (-9.2051, -126.1776) (-9.2097, -126.1597) (-9.219, -126.1241) (-9.2327, -126.0705) (-9.2509, -125.9991) (-9.2733, -125.9099) (-9.2954, -125.8206) (-9.3172, -125.7314) (-9.3387, -125.6421) (-9.3599, -125.5528) (-9.3808, -125.4635) (-9.4014, -125.3742) (-9.4217, -125.285) (-9.4416, -125.1957) (-9.4612, -125.1064) (-9.4805, -125.0171) (-9.4995, -124.9278) (-9.5181, -124.8385) (-9.5365, -124.7492) (-9.5545, -124.6599) (-9.5721, -124.5706) (-9.5894, -124.4813) (-9.6064, -124.3921) (-9.6231, -124.3028) (-9.6394, -124.2135) (-9.6553, -124.1242) (-9.6709, -124.035) (-9.6861, -123.9457) (-9.701, -123.8565) (-9.7156, -123.7672) (-9.7297, -123.678) (-9.7435, -123.5888) (-9.7569, -123.4996) (-9.77, -123.4104) (-9.7827, -123.3212) (-9.7949, -123.2321) (-9.8068, -123.1429) (-9.8183, -123.0538) (-9.8294, -122.9647) (-9.8401, -122.8756) (-9.8504, -122.7866) (-9.8603, -122.6975) (-9.869, -122.6158) (-9.8755, -122.5519) (-9.8801, -122.5057) (-9.8828, -122.4774) (-9.8838, -122.4669) knots -1 -1 -1 -1 -1 -1 -0.985714 -0.971429 -0.957143 -0.942857 -0.928571 -0.914286 -0.9 -0.885714 -0.871429 -0.857143 -0.842857 -0.828571 -0.814286 -0.8 -0.785714 -0.771429 -0.757143 -0.742857 -0.728571 -0.714286 -0.7 -0.685714 -0.671429 -0.657143 -0.642857 -0.628571 -0.614286 -0.6 -0.585714 -0.571429 -0.557143 -0.542857 -0.528571 -0.514286 -0.5 -0.485714 -0.471429 -0.457143 -0.442857 -0.428571 -0.414286 -0.405839 -0.405839 -0.405839 -0.405839 -0.405839 -0.405839
  arc A138 (-11.181, -122.2329) -> (-9.8838, -122.4669) centre (2.0032, -52.8695) ccw
  spline S139 degree 5 poles (-11.181, -122.2329) (-11.1856, -122.2424) (-11.1981, -122.2679) (-11.2185, -122.3096) (-11.2469, -122.3672) (-11.2837, -122.4407) (-11.324, -122.5207) (-11.3648, -122.6005) (-11.406, -122.6803) (-11.4475, -122.7599) (-11.4894, -122.8394) (-11.5317, -122.9187) (-11.5744, -122.998) (-11.6174, -123.0771) (-11.6608, -123.1561) (-11.7046, -123.235) (-11.7487, -123.3138) (-11.7931, -123.3924) (-11.8379, -123.4709) (-11.883, -123.5494) (-11.9285, -123.6277) (-11.9743, -123.7058) (-12.0205, -123.7839) (-12.0669, -123.8618) (-12.1137, -123.9397) (-12.1608, -124.0174) (-12.2083, -124.095) (-12.256, -124.1725) (-12.3041, -124.2499) (-12.3524, -124.3271) (-12.4011, -124.4043) (-12.4501, -124.4813) (-12.4994, -124.5582) (-12.549, -124.635) (-12.5989, -124.7117) (-12.6491, -124.7883) (-12.6995, -124.8648) (-12.7503, -124.9411) (-12.8014, -125.0174) (-12.8527, -125.0935) (-12.9043, -125.1695) (-12.9562, -125.2454) (-13.0084, -125.3212) (-13.0504, -125.3817) (-13.082, -125.4271) (-13.1031, -125.4573) (-13.1137, -125.4724) knots 0.405839 0.405839 0.405839 0.405839 0.405839 0.405839 0.414286 0.428571 0.442857 0.457143 0.471429 0.485714 0.5 0.514286 0.528571 0.542857 0.557143 0.571429 0.585714 0.6 0.614286 0.628571 0.642857 0.657143 0.671429 0.685714 0.7 0.714286 0.728571 0.742857 0.757143 0.771429 0.785714 0.8 0.814286 0.828571 0.842857 0.857143 0.871429 0.885714 0.9 0.914286 0.928571 0.942857 0.957143 0.971429 0.985714 1 1 1 1 1 1
  arc A139 (-14.4063, -125.1912) -> (-13.1137, -125.4724) centre (2.0032, -52.8695) ccw
  spline S140 degree 5 poles (-14.4063, -125.1912) (-14.4096, -125.1731) (-14.4163, -125.1368) (-14.4262, -125.0824) (-14.4392, -125.0099) (-14.4552, -124.9193) (-14.4709, -124.8287) (-14.4863, -124.7381) (-14.5014, -124.6475) (-14.5162, -124.557) (-14.5306, -124.4664) (-14.5448, -124.3759) (-14.5586, -124.2854) (-14.5721, -124.1949) (-14.5853, -124.1045) (-14.5982, -124.014) (-14.6108, -123.9236) (-14.623, -123.8332) (-14.6349, -123.7428) (-14.6465, -123.6525) (-14.6577, -123.5622) (-14.6686, -123.4719) (-14.6792, -123.3816) (-14.6894, -123.2914) (-14.6993, -123.2012) (-14.7089, -123.111) (-14.718, -123.0208) (-14.7269, -122.9307) (-14.7354, -122.8406) (-14.7435, -122.7506) (-14.7513, -122.6606) (-14.7586, -122.5706) (-14.7657, -122.4807) (-14.7723, -122.3908) (-14.7786, -122.3009) (-14.7845, -122.2111) (-14.79, -122.1214) (-14.7951, -122.0317) (-14.7998, -121.942) (-14.8041, -121.8524) (-14.8081, -121.7628) (-14.8116, -121.6733) (-14.8144, -121.5911) (-14.8163, -121.5269) (-14.8176, -121.4806) (-14.8183, -121.4521) (-14.8186, -121.4416) knots -1 -1 -1 -1 -1 -1 -0.985714 -0.971429 -0.957143 -0.942857 -0.928571 -0.914286 -0.9 -0.885714 -0.871429 -0.857143 -0.842857 -0.828571 -0.814286 -0.8 -0.785714 -0.771429 -0.757143 -0.742857 -0.728571 -0.714286 -0.7 -0.685714 -0.671429 -0.657143 -0.642857 -0.628571 -0.614286 -0.6 -0.585714 -0.571429 -0.557143 -0.542857 -0.528571 -0.514286 -0.5 -0.485714 -0.471429 -0.457143 -0.442857 -0.428571 -0.414286 -0.405839 -0.405839 -0.405839 -0.405839 -0.405839 -0.405839
  arc A140 (-16.0958, -121.1156) -> (-14.8186, -121.4416) centre (2.0032, -52.8695) ccw
  spline S141 degree 5 poles (-16.0958, -121.1156) (-16.101, -121.1247) (-16.1153, -121.1493) (-16.1386, -121.1894) (-16.1711, -121.2448) (-16.213, -121.3156) (-16.2589, -121.3925) (-16.3053, -121.4692) (-16.352, -121.5458) (-16.3991, -121.6222) (-16.4466, -121.6985) (-16.4945, -121.7747) (-16.5427, -121.8507) (-16.5913, -121.9265) (-16.6402, -122.0022) (-16.6895, -122.0778) (-16.7391, -122.1532) (-16.789, -122.2285) (-16.8393, -122.3036) (-16.8899, -122.3786) (-16.9409, -122.4535) (-16.9921, -122.5282) (-17.0437, -122.6028) (-17.0956, -122.6772) (-17.1478, -122.7515) (-17.2004, -122.8257) (-17.2532, -122.8997) (-17.3064, -122.9736) (-17.3598, -123.0473) (-17.4136, -123.1209) (-17.4677, -123.1944) (-17.522, -123.2678) (-17.5767, -123.341) (-17.6316, -123.414) (-17.6868, -123.487) (-17.7424, -123.5598) (-17.7982, -123.6325) (-17.8542, -123.705) (-17.9106, -123.7774) (-17.9672, -123.8497) (-18.0242, -123.9218) (-18.0814, -123.9938) (-18.1388, -124.0657) (-18.185, -124.1231) (-18.2198, -124.166) (-18.243, -124.1947) (-18.2546, -124.209) knots 0.405839 0.405839 0.405839 0.405839 0.405839 0.405839 0.414286 0.428571 0.442857 0.457143 0.471429 0.485714 0.5 0.514286 0.528571 0.542857 0.557143 0.571429 0.585714 0.6 0.614286 0.628571 0.642857 0.657143 0.671429 0.685714 0.7 0.714286 0.728571 0.742857 0.757143 0.771429 0.785714 0.8 0.814286 0.828571 0.842857 0.857143 0.871429 0.885714 0.9 0.914286 0.928571 0.942857 0.957143 0.971429 0.985714 1 1 1 1 1 1
  arc A141 (-19.5238, -123.8363) -> (-18.2546, -124.209) centre (2.0032, -52.8695) ccw
  spline S142 degree 5 poles (-19.5238, -123.8363) (-19.5259, -123.818) (-19.53, -123.7813) (-19.536, -123.7264) (-19.5438, -123.6531) (-19.5533, -123.5616) (-19.5625, -123.4701) (-19.5713, -123.3787) (-19.5799, -123.2872) (-19.5882, -123.1959) (-19.5962, -123.1045) (-19.6038, -123.0132) (-19.6112, -122.9219) (-19.6182, -122.8307) (-19.6249, -122.7396) (-19.6313, -122.6484) (-19.6374, -122.5573) (-19.6431, -122.4663) (-19.6486, -122.3753) (-19.6537, -122.2844) (-19.6584, -122.1935) (-19.6629, -122.1026) (-19.667, -122.0118) (-19.6707, -121.9211) (-19.6742, -121.8304) (-19.6772, -121.7398) (-19.68, -121.6492) (-19.6824, -121.5587) (-19.6844, -121.4682) (-19.6861, -121.3778) (-19.6874, -121.2875) (-19.6884, -121.1972) (-19.689, -121.107) (-19.6892, -121.0169) (-19.689, -120.9268) (-19.6885, -120.8368) (-19.6876, -120.7469) (-19.6863, -120.6571) (-19.6846, -120.5673) (-19.6825, -120.4776) (-19.68, -120.388) (-19.6771, -120.2984) (-19.6741, -120.2163) (-19.6715, -120.1521) (-19.6694, -120.1058) (-19.6681, -120.0774) (-19.6676, -120.0668) knots -1 -1 -1 -1 -1 -1 -0.985714 -0.971429 -0.957143 -0.942857 -0.928571 -0.914286 -0.9 -0.885714 -0.871429 -0.857143 -0.842857 -0.828571 -0.814286 -0.8 -0.785714 -0.771429 -0.757143 -0.742857 -0.728571 -0.714286 -0.7 -0.685714 -0.671429 -0.657143 -0.642857 -0.628571 -0.614286 -0.6 -0.585714 -0.571429 -0.557143 -0.542857 -0.528571 -0.514286 -0.5 -0.485714 -0.471429 -0.457143 -0.442857 -0.428571 -0.414286 -0.405839 -0.405839 -0.405839 -0.405839 -0.405839 -0.405839
  arc A142 (-20.9183, -119.6505) -> (-19.6676, -120.0668) centre (2.0032, -52.8695) ccw
  spline S143 degree 5 poles (-20.9183, -119.6505) (-20.9242, -119.6593) (-20.9402, -119.6828) (-20.9663, -119.7211) (-21.0026, -119.7741) (-21.0494, -119.8417) (-21.1008, -119.9151) (-21.1525, -119.9883) (-21.2046, -120.0614) (-21.257, -120.1343) (-21.3098, -120.207) (-21.363, -120.2795) (-21.4165, -120.3519) (-21.4704, -120.4241) (-21.5246, -120.4961) (-21.5791, -120.5679) (-21.634, -120.6396) (-21.6891, -120.7112) (-21.7447, -120.7825) (-21.8005, -120.8537) (-21.8566, -120.9247) (-21.9131, -120.9956) (-21.9699, -121.0663) (-22.027, -121.1369) (-22.0844, -121.2072) (-22.1421, -121.2775) (-22.2001, -121.3475) (-22.2584, -121.4174) (-22.3169, -121.4872) (-22.3758, -121.5568) (-22.435, -121.6262) (-22.4944, -121.6955) (-22.5542, -121.7646) (-22.6142, -121.8336) (-22.6745, -121.9024) (-22.735, -121.971) (-22.7959, -122.0395) (-22.857, -122.1079) (-22.9184, -122.1761) (-22.98, -122.2441) (-23.042, -122.312) (-23.1041, -122.3798) (-23.1666, -122.4474) (-23.2168, -122.5013) (-23.2545, -122.5417) (-23.2797, -122.5686) (-23.2923, -122.582) knots 0.405839 0.405839 0.405839 0.405839 0.405839 0.405839 0.414286 0.428571 0.442857 0.457143 0.471429 0.485714 0.5 0.514286 0.528571 0.542857 0.557143 0.571429 0.585714 0.6 0.614286 0.628571 0.642857 0.657143 0.671429 0.685714 0.7 0.714286 0.728571 0.742857 0.757143 0.771429 0.785714 0.8 0.814286 0.828571 0.842857 0.857143 0.871429 0.885714 0.9 0.914286 0.928571 0.942857 0.957143 0.971429 0.985714 1 1 1 1 1 1
  arc A143 (-24.5317, -122.1198) -> (-23.2923, -122.582) centre (2.0032, -52.8695) ccw
  spline S144 degree 5 poles (-24.5317, -122.1198) (-24.5324, -122.1014) (-24.5339, -122.0645) (-24.536, -122.0093) (-24.5385, -121.9356) (-24.5415, -121.8437) (-24.5441, -121.7518) (-24.5464, -121.6599) (-24.5485, -121.5681) (-24.5502, -121.4764) (-24.5516, -121.3847) (-24.5528, -121.2931) (-24.5536, -121.2015) (-24.5541, -121.11) (-24.5543, -121.0186) (-24.5542, -120.9272) (-24.5537, -120.836) (-24.553, -120.7447) (-24.5519, -120.6536) (-24.5505, -120.5625) (-24.5488, -120.4715) (-24.5467, -120.3806) (-24.5443, -120.2897) (-24.5416, -120.199) (-24.5385, -120.1083) (-24.5352, -120.0176) (-24.5314, -119.9271) (-24.5273, -119.8366) (-24.5229, -119.7463) (-24.5182, -119.656) (-24.513, -119.5658) (-24.5075, -119.4757) (-24.5017, -119.3857) (-24.4955, -119.2958) (-24.4889, -119.2059) (-24.482, -119.1162) (-24.4746, -119.0266) (-24.4669, -118.937) (-24.4588, -118.8476) (-24.4504, -118.7583) (-24.4415, -118.6691) (-24.4322, -118.58) (-24.4233, -118.4982) (-24.4161, -118.4344) (-24.4108, -118.3884) (-24.4074, -118.3601) (-24.4062, -118.3496) knots -1 -1 -1 -1 -1 -1 -0.985714 -0.971429 -0.957143 -0.942857 -0.928571 -0.914286 -0.9 -0.885714 -0.871429 -0.857143 -0.842857 -0.828571 -0.814286 -0.8 -0.785714 -0.771429 -0.757143 -0.742857 -0.728571 -0.714286 -0.7 -0.685714 -0.671429 -0.657143 -0.642857 -0.628571 -0.614286 -0.6 -0.585714 -0.571429 -0.557143 -0.542857 -0.528571 -0.514286 -0.5 -0.485714 -0.471429 -0.457143 -0.442857 -0.428571 -0.414286 -0.405839 -0.405839 -0.405839 -0.405839 -0.405839 -0.405839
  arc A144 (-25.624, -117.8452) -> (-24.4062, -118.3496) centre (2.0032, -52.8695) ccw
  spline S145 degree 5 poles (-25.624, -117.8452) (-25.6305, -117.8535) (-25.6481, -117.8758) (-25.6769, -117.9122) (-25.7169, -117.9624) (-25.7684, -118.0265) (-25.8249, -118.096) (-25.8817, -118.1654) (-25.9389, -118.2346) (-25.9964, -118.3035) (-26.0542, -118.3723) (-26.1124, -118.4408) (-26.171, -118.5092) (-26.2298, -118.5774) (-26.289, -118.6453) (-26.3486, -118.7131) (-26.4084, -118.7807) (-26.4685, -118.8481) (-26.529, -118.9153) (-26.5898, -118.9824) (-26.6509, -119.0492) (-26.7122, -119.1159) (-26.7739, -119.1823) (-26.8359, -119.2486) (-26.8982, -119.3147) (-26.9607, -119.3807) (-27.0236, -119.4464) (-27.0867, -119.512) (-27.1501, -119.5774) (-27.2138, -119.6426) (-27.2778, -119.7076) (-27.342, -119.7725) (-27.4065, -119.8372) (-27.4713, -119.9017) (-27.5363, -119.966) (-27.6017, -120.0302) (-27.6672, -120.0942) (-27.7331, -120.158) (-27.7992, -120.2216) (-27.8655, -120.2851) (-27.9321, -120.3484) (-27.999, -120.4115) (-28.0661, -120.4745) (-28.12, -120.5247) (-28.1605, -120.5623) (-28.1876, -120.5873) (-28.2011, -120.5999) knots 0.405839 0.405839 0.405839 0.405839 0.405839 0.405839 0.414286 0.428571 0.442857 0.457143 0.471429 0.485714 0.5 0.514286 0.528571 0.542857 0.557143 0.571429 0.585714 0.6 0.614286 0.628571 0.642857 0.657143 0.671429 0.685714 0.7 0.714286 0.728571 0.742857 0.757143 0.771429 0.785714 0.8 0.814286 0.828571 0.842857 0.857143 0.871429 0.885714 0.9 0.914286 0.928571 0.942857 0.957143 0.971429 0.985714 1 1 1 1 1 1
  arc A145 (-29.4044, -120.0504) -> (-28.2011, -120.5999) centre (2.0032, -52.8695) ccw
  spline S146 degree 5 poles (-29.4044, -120.0504) (-29.4038, -120.0319) (-29.4026, -119.9951) (-29.4007, -119.9398) (-29.398, -119.8662) (-29.3944, -119.7743) (-29.3905, -119.6824) (-29.3862, -119.5906) (-29.3817, -119.4989) (-29.3769, -119.4073) (-29.3718, -119.3157) (-29.3664, -119.2242) (-29.3607, -119.1329) (-29.3546, -119.0416) (-29.3483, -118.9504) (-29.3417, -118.8593) (-29.3347, -118.7682) (-29.3275, -118.6773) (-29.3199, -118.5865) (-29.312, -118.4957) (-29.3038, -118.4051) (-29.2952, -118.3145) (-29.2864, -118.2241) (-29.2772, -118.1337) (-29.2677, -118.0435) (-29.2578, -117.9533) (-29.2477, -117.8633) (-29.2371, -117.7734) (-29.2263, -117.6835) (-29.2151, -117.5938) (-29.2035, -117.5042) (-29.1916, -117.4147) (-29.1794, -117.3254) (-29.1668, -117.2361) (-29.1538, -117.147) (-29.1405, -117.058) (-29.1268, -116.9691) (-29.1127, -116.8803) (-29.0982, -116.7917) (-29.0834, -116.7032) (-29.0682, -116.6149) (-29.0526, -116.5266) (-29.0379, -116.4458) (-29.0261, -116.3826) (-29.0175, -116.3371) (-29.0122, -116.3091) (-29.0102, -116.2987) knots -1 -1 -1 -1 -1 -1 -0.985714 -0.971429 -0.957143 -0.942857 -0.928571 -0.914286 -0.9 -0.885714 -0.871429 -0.857143 -0.842857 -0.828571 -0.814286 -0.8 -0.785714 -0.771429 -0.757143 -0.742857 -0.728571 -0.714286 -0.7 -0.685714 -0.671429 -0.657143 -0.642857 -0.628571 -0.614286 -0.6 -0.585714 -0.571429 -0.557143 -0.542857 -0.528571 -0.514286 -0.5 -0.485714 -0.471429 -0.457143 -0.442857 -0.428571 -0.414286 -0.405839 -0.405839 -0.405839 -0.405839 -0.405839 -0.405839
  arc A146 (-30.1889, -115.7087) -> (-29.0102, -116.2987) centre (2.0032, -52.8695) ccw